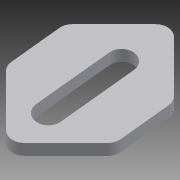
# Autodesk Inventor part: hph_D_001
Saved by Autodesk Inventor 2014 (Build 180170000, 170)
## iProperties
Created: 2014-03-22
Part Number: hph_D_001
Material: Generic
Document SubType Name: Modeling
Designer: stephenholtz
Density: 1 g/cm^3
Appearance: Default
Mass: 0.241552 g
Surface Area: 4.29018 cm^2
Volume: 0.241552 cm^3
Description: Laser Cut Grade 5 Titanium
Author: stephenholtz
Revision Number: 1
Autodesk Inventor part; units mm, degrees
ref_plane "YZ Plane" through (0, 0, 0) normal (1, 0, 0) x (0, 1, 0)
ref_plane "XZ Plane" through (0, 0, 0) normal (0, 1, 0) x (-1, 0, 0)
ref_plane "XY Plane" through (0, 0, 0) normal (0, 0, 1) x (1, 0, 0)
sketch "Sketch2" plane through (0, 0, 0) normal (0, 0, 1) x (1, 0, 0)
  line L0 (-4.7625, -4.7625) -> (4.7625, -4.7625)
  line L1 (4.7625, -4.7625) -> (4.7625, 4.7625)
  line L2 (4.7625, 4.7625) -> (-4.7625, 4.7625)
  line L3 (-4.7625, 4.7625) -> (-4.7625, -4.7625)
  line L4 (-4.7625, -4.7625) -> (4.7625, 4.7625) construction
  line L5 (4.7625, -4.7625) -> (-4.7625, 4.7625) construction
  line L6 (-4.7625, 4.7625) -> (4.7625, -4.7625)
  line L7 (4.7625, -4.7625) -> (-0.3562, -9.8812)
  line L8 (-0.3562, -9.8812) -> (-9.8812, -0.3562)
  line L9 (-9.8812, -0.3562) -> (-4.7625, 4.7625)
  line L10 (-9.8812, -0.3562) -> (-9.8812, -9.8812)
  line L11 (-9.8812, -9.8812) -> (-0.3562, -9.8812)
  line L12 (-0.3562, -9.8812) -> (-0.3562, -0.3562)
  line L13 (-0.3562, -0.3562) -> (-9.8812, -0.3562)
  line L14 (-9.8812, -0.3562) -> (-0.3562, -9.8812) construction
  line L15 (-9.8812, -9.8812) -> (-0.3562, -0.3562) construction
  point P0 (0, 0)
  point P1 (-5.1187, -5.1187)
  point P2 (-5.1187, -5.1187)
  dimension "clip_edge" = 9.525
  dimension "d1" = 9.525
  dimension "d2" = 7.239
  dimension "d39" = 9.525
  dimension "d40" = 9.525
  constraints: 32 end point, 7 equal length, 6 midpoint, 3 perpendicular, 1 horizontal
  measures "clip_edge" distance of L0.end L1.end
  measures "d1" distance of L0.start L0.end
  measures "d2" distance of L8.end L2.end
  measures "d39" distance of L12.end L10.start
  measures "d40" distance of L10.start L10.end
extrude "Extrusion1" add sketch "Sketch2" along normal blind 1.5875
sketch "Sketch3" plane through (0, 0, 0) normal (0, 0, -1) x (-1, 0, 0)
  line L0 (6.1855, -6.1855) -> (-0.1905, 0.1905)
  line L1 (0.3562, -9.8812) -> (-4.7625, -4.7625) construction
  line L2 (-4.7625, 4.7625) -> (5.1187, -5.1187) construction
  line L3 (9.8812, -0.3562) -> (0.3562, -9.8812) construction
  line L4 (-4.7625, 4.7625) -> (4.7625, 4.7625) projected
  line L5 (6.1855, -6.1855) -> (-0.1905, 0.1905) construction
  line L6 (7.2631, -5.1079) -> (0.8871, 1.2681)
  line L7 (-1.2681, -0.8871) -> (5.1079, -7.2631)
  arc A0 (5.1079, -7.2631) -> (7.2631, -5.1079) centre (6.1855, -6.1855) ccw
  arc A1 (0.8871, 1.2681) -> (-1.2681, -0.8871) centre (-0.1905, 0.1905) ccw
  point P0 (0, 0)
  point P1 (2.9975, -2.9975)
  dimension "d5" = 9.017
  dimension "d6" = 4.572
  dimension "d31" = 3.048
  constraints: 14 end point, 4 point on circle, 4 tangent, 3 parallel, 2 centre point, 2 collinear, 2 midpoint, 1 coincident
  measures "d5" distance of L0.start L0.end
  measures "d6" distance from line of L4 L0.end
  measures "d31" distance between parallel lines of L6 L7
extrude "Extrusion7" cut sketch "Sketch3" against normal through all
fillet "Fillet13" radius 1.5875 6 edges at (-4.7625, 4.7625, 0.7937) (-9.8812, -0.3562, 0.7937) (-9.8812, -9.8812, 0.7937) (4.7625, -4.7625, 0.7937) (4.7625, 4.7625, 0.7937) (-0.3562, -9.8812, 0.7937)
equation "\"d1\" = clip_edge"
body "Solid1"
